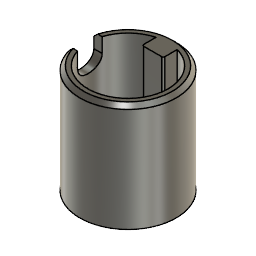
Yarbo Wall Mount Bushing (Autodesk Fusion 360 design; units mm, degrees)
Autodesk Fusion 360 part; units mm, degrees
note: some values were not read from the file. Chosen so that the rebuilt part matches the saved one: which face or edge a step refers to. Set by a fixed rule: which sketch regions a step uses.
sketch "Sketch1" plane through (0, 0, 0) normal (0, 0, 1) x (1, 0, 0)
  circle A0 centre (0, 0) radius 12.5
  circle A1 centre (0, 0) radius 10.4
  line L0 (2.75, 10.0298) -> (2.75, 6.4)
  line L1 (0, 2.5) -> (0, 20) construction
  line L2 (-2.75, 10.0298) -> (-2.75, 6.4)
  line L3 (2.75, 6.4) -> (-2.75, 6.4)
  dimension "d1" = 25
  dimension "d2" = 20.8
  dimension "d3" = 5.5
  dimension "d5" = 4
  constraint coincident A0.centre A1.centre
  constraint concentric A0 A1
  constraint coincident A1 L0.start
  constraint vertical L0
  constraint symmetric L0.start L1 L2.start
  constraint symmetric L0.end L1 L2.end
  measures "d1" diameter of A0
  measures "d2" diameter of A1
  measures "d3" distance of L0 L2
  measures "d5" distance of A1 L3
extrude "Extrude1" add sketch "Sketch1" along normal blind 28 contours A0 | A1 L0 L2 L3 picked at (0, 7.7333)
sketch "Sketch2" plane through (0, 0, 0) normal (1, 0, 0) x (0, 1, 0)
  line L0 (0, 0) -> (0, 24.2) construction
  circle A0 centre (0, 24.2) radius 3.2
  line L1 (-3.2, 24.2) -> (-3.2, 28)
  line L2 (3.2, 24.2) -> (3.2, 28)
  line L3 (12.5, 28) -> (-12.5, 28)
  dimension "d8" = 6.4
  dimension "d9" = 21
  constraint coincident L0.start origin
  constraint vertical L0
  constraint coincident L0.end A0.centre
  constraint coincident A0 L1.start
  constraint parallel L0 L1
  constraint coincident A0 L2.start
  constraint tangent A0 L2
  constraint tangent A0 L1
  constraint vertical L2
  constraint coincident L3 L1.end
  constraint coincident L3 L2.end
  measures "d8" diameter of A0
  measures "d9" distance of L0.start A0
extrude "Extrude2" cut sketch "Sketch2" against normal blind 20.652
chamfer "Chamfer1" distance 1 angle 45 2 edges at (1.6135, -12.3954, 28) (1.6135, 12.3954, 28)
fillet "Fillet1" radius 0.4 2 edges at (2.75, 6.4, 14) (-2.75, 6.4, 14)
named bodies: "Yarbo Wall Mount Bushing"
